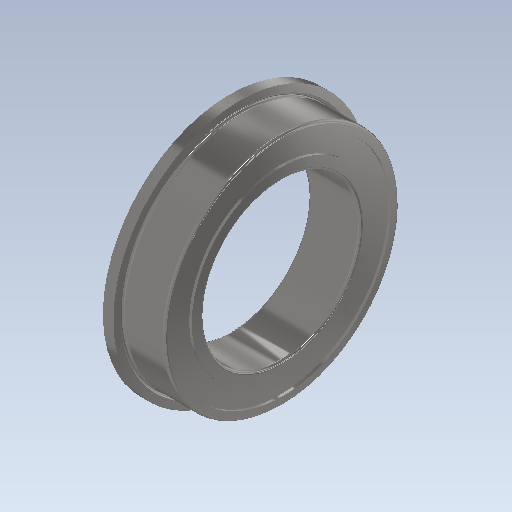
# Autodesk Inventor part: FL6701ZZ
Saved by Autodesk Inventor 2021 (Build 250183000, 183)
## iProperties
Category: PARTsolutions
Company: MISUMI
Part Number: FL6701ZZ
Material: 鉄、鋳鉄
Catalog Web Link: www.cadenas.de
Description: FL6 _ _ ZZ, FL6 _ _ AZZ, SFL6 _ _ ZZ, SFL6 _ _ AZZ, MFL1 _ _ ZZ, SMFL1 _ _ ZZ-Flanged Ball Bearings (Small Diameter, Deep Groove) - Double Shield Type
Vendor: MISUMI
Document SubType Name: Modeling
Designer: partserver
Manufacturer: MISUMI
Mass: 4.05488 g
Surface Area: 8.09255 cm^2
Volume: 0.567116 cm^3
Density: 7.15 g/cm^3
Appearance: 鋼 - つや出し
PSOL_IDENT_0: {$CADENAS_DATA\23d-libs\misumi\metric\12_bearing_holders\sfl608zz.prj},231 {VTYP=3D},{NB=FL6701ZZ},{
PSOL_IDENT_1: LINA=FL6701ZZ},{NN=FL6 _ _ ZZ, FL6 _ _ AZZ, SFL6 _ _ ZZ, SFL6 _ _ AZZ, MFL1 _ _ ZZ, SMFL1 _ _ ZZ},{D
PSOL_IDENT_2: ATE=09.09.2019 15:26:56},{GEOMDATE=16.08.2017 04:27:24},{VERSION=},{LINEID=350},{WBVAR=MAT},{WBNUMER
PSOL_IDENT_3: IC=}  {NB=FL6701ZZ},{LINA=FL6701ZZ},{KT=DUMMY},{PN=FL6701ZZ},{MAT=},{MAT1= '', '52100 Bearing Steel'
PSOL_IDENT_4: , 'S', '440C Stainless Steel'},{BN=6701ZZ},{DD=12.0},{AA=3.6000},{BB=0.6500},{C1=0.9300},{D=18},{B=4
PSOL_IDENT_5: .0},{D1=19.5},{C=0.8},{RR=0.20},{CR=926},{COR=530},{CRS=926},{CRSS=787},{CORS=530},{CORSS=424},{DS=1
PSOL_IDENT_6: 2.40},{R=0.20},{MASS=3.4},{MAT11=1},{MMMM=}
NB: FL6701ZZ
NN: FL6 _ _ ZZ, FL6 _ _ AZZ, SFL6 _ _ ZZ, SFL6 _ _ AZZ, MFL1 _ _ ZZ, SMFL1 _ _ ZZ
NT: Flanged Ball Bearings (Small Diameter, Deep Groove) - Double Shield Type
NBSYN: $PN.
LINA: FL6701ZZ
CATALOG: Misumi
PN: FL6701ZZ
MAT: 52100 Bearing Steel
BN: 6701ZZ
DD: 12
D: 18
B: 4
D1: 0
C: 0.8
RR: 0.2
CR: 926
COR: 530
DS: 12.4
R: 0.2
MASS: 3.4
SUPPLIER: MISUMI
ARTICLENO: FL6701ZZ
BOMINFO: FL6701ZZ
CREATOR: CADENAS GmbH
Title: FL6701ZZ
Author: Cadenas PARTsolutions
Comments: Flanged Ball Bearings (Small Diameter, Deep Groove) - Double Shield Type
Autodesk Inventor part; units mm, degrees
sketch "Sketch_1" plane through (0, 0, 0) normal (0, 0, 1) x (1, 0, 0)
  line L0 (18, 0) -> (-18, 0)
  arc A0 (0, 6.2) -> (0.2, 6) centre (0.2, 6.2) ccw
  line L1 (0.2, 6) -> (3.8, 6)
  arc A1 (3.8, 6) -> (4, 6.2) centre (3.8, 6.2) ccw
  line L2 (4, 6.2) -> (4, 6.93)
  line L3 (4, 6.93) -> (3.8, 6.93)
  line L4 (3.8, 6.93) -> (3.8, 8.35)
  line L5 (3.8, 8.35) -> (4, 8.35)
  line L6 (4, 8.35) -> (4, 9.75)
  line L7 (4, 9.75) -> (3.2, 9.75)
  line L8 (3.2, 9.75) -> (3.2, 9.2)
  arc A2 (3, 9) -> (3.2, 9.2) centre (3.2, 9) ccw
  line L9 (3, 9) -> (0.2, 9)
  arc A3 (0.2, 9) -> (0, 8.8) centre (0.2, 8.8) ccw
  line L10 (0, 8.8) -> (0, 8.35)
  line L11 (0, 8.35) -> (0.2, 8.35)
  line L12 (0.2, 8.35) -> (0.2, 6.93)
  line L13 (0.2, 6.93) -> (0, 6.93)
  line L14 (0, 6.93) -> (0, 6.2)
  constraints: 30 end point, 8 point on circle, 4 centre point
revolve "Revolution1" add sketch "Sketch_1" angle 360 about axis through (18, 0, 0) along (1, 0, 0)
ref_plane "to_housing_XY" through (0, 0, 0) normal (1, 0, 0) x (0, 0, -1)
ref_plane "to_housing_YZ" through (0, 0, 0) normal (0, 0, -1) x (0, 1, 0)
ref_plane "to_housing_ZX" through (0, 0, 0) normal (0, 1, 0) x (1, 0, 0)
body "Solid1"
